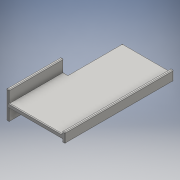
# Autodesk Inventor part: halfPartition
Saved by Autodesk Inventor 2016 (Build 200138000, 138)
## iProperties
Created: 2017-04-06
Part Number: halfPartition
Material: 一般
Document SubType Name: Modeling
Designer: Daisuke
Density: 1 g/cm^3
Appearance: 既定
Author: Daisuke
## iProperties of the stored document halfPartition_3D プリント.ipt
Created: 2017-04-06
Part Number: halfPartition_3D プリント
Material: 一般
Document SubType Name: Modeling
Designer: Daisuke
Density: 1 g/cm^3
Appearance: 既定
Author: Daisuke
Autodesk Inventor part; units mm, degrees
ref_plane "YZ Plane" through (0, 0, 0) normal (1, 0, 0) x (0, 1, 0)
ref_plane "XZ Plane" through (0, 0, 0) normal (0, 1, 0) x (-1, 0, 0)
ref_plane "XY Plane" through (0, 0, 0) normal (0, 0, 1) x (1, 0, 0)
sketch "スケッチ1" plane through (0, 0, 0) normal (0, 1, 0) x (-1, 0, 0)
  line L0 (0, 0) -> (-40, 0)
  line L1 (-40, 0) -> (-40, -3)
  line L2 (-40, -3) -> (0, -3)
  line L3 (0, -3) -> (0, 0)
  line L4 (-39, 2) -> (-41, 2)
  line L5 (-41, 2) -> (-41, -5)
  line L6 (-41, -5) -> (-39, -5)
  line L7 (-39, -5) -> (-39, 2)
  line L8 (-39, 2) -> (-41, -5) construction
  line L9 (-41, 2) -> (-39, -5) construction
  line L10 (1, 8.5) -> (-1, 8.5)
  line L11 (-1, 8.5) -> (-1, -11.5)
  line L12 (-1, -11.5) -> (1, -11.5)
  line L13 (1, -11.5) -> (1, 8.5)
  line L14 (1, 8.5) -> (-1, -11.5) construction
  line L15 (-1, 8.5) -> (1, -11.5) construction
  point P0 (-40, -1.5)
  point P1 (0, -1.5)
  dimension "d1" = 40
  dimension "d2" = 3
  dimension "d3" = 2
  dimension "d4" = 7
  dimension "d5" = 2
  dimension "d6" = 20
  constraints: 32 end point, 6 midpoint, 6 parallel, 3 horizontal, 3 perpendicular
  measures "d1" distance of L2.end L1.end
  measures "d2" distance of L1.end L0.end
  measures "d3" distance of L6.end L5.end
  measures "d4" distance of L5.end L4.end
  measures "d5" distance of L12.end L11.end
  measures "d6" distance of L11.end L10.end
extrude "押し出し1" add sketch "スケッチ1" along normal blind 78
sketch "スケッチ2" plane through (0, 78, 0) normal (0, 1, 0) x (1, 0, 0)
  line L0 (1, 3) -> (1, 11.5) projected
  line L1 (-1, -8.5) -> (1, -8.5)
  line L2 (1, -8.5) -> (1, 11.5)
  line L3 (1, 11.5) -> (-1, 11.5)
  line L4 (-1, 11.5) -> (-1, -8.5)
  line L5 (1, 0) -> (39, 0) projected
  line L6 (1, 0) -> (4.2, 0)
  line L7 (4.2, 0) -> (4.2, 3)
  line L8 (4.2, 3) -> (1, 3)
  line L9 (1, 3) -> (1, 0)
  point P0 (0, 0)
  dimension "d9" = 2
  dimension "d10" = 20
  dimension "d11" = 3.2
  dimension "d12" = 3
  constraints: 16 end point, 4 parallel, 2 horizontal, 2 perpendicular
  measures "d9" distance of L3.end L0.end
  measures "d10" distance of L0.end L1.end
  measures "d11" distance of L8.end L7.end
  measures "d12" distance of L7.end L6.end
extrude "押し出し2" cut sketch "スケッチ2" against normal blind 39
fillet "フィレット1" radius 0.5 38 edges at (1, 0, 4.25) (-1, 0, -1.5) (1, 19.5, 8.5) (0, 0, -11.5) (1, 0, -7.25) (20, 0, 0) (20, 0, -3) (0, 0, 8.5) (41, 0, -1.5) (40, 0, 2) (39, 39, 0) (40, 0, -5) (39, 0, 1) (39, 0, -4) (41, 39, -5) (39, 39, -5) (41, 39, 2) (41, 78, -1.5) (40, 78, -5) (21.6, 78, -3) (4.2, 58.5, 0) (2.6, 39, 0) (1, 39, 4.25) (0, 39, 8.5) (-1, 19.5, 8.5) (39, 39, 2) (21.6, 78, 0) (40, 78, 2) (39, 78, 1) (4.2, 78, -1.5) (4.2, 58.5, -3) (39, 78, -4) (-1, 19.5, -11.5) (1, 19.5, -11.5) (0, 39, -11.5) (1, 39, -7.25) (-1, 39, -1.5) (2.6, 39, -3)
